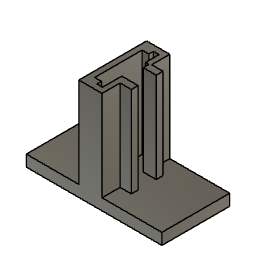
Camera_holder (Autodesk Fusion 360 design; units mm, degrees)
Autodesk Fusion 360 part; units mm, degrees
sketch "Esquisse1" plane through (0, 0, 0) normal (0, 0, 1) x (1, 0, 0)
  line L0 (-29.5177, 14.6047) -> (30.4823, 14.6047)
  line L1 (30.4823, 14.6047) -> (30.4823, -15.3953)
  line L2 (30.4823, -15.3953) -> (-29.5177, -15.3953)
  line L3 (-29.5177, -15.3953) -> (-29.5177, 14.6047)
  dimension "d1" = 60
  dimension "d2" = 30
  constraint horizontal L0
  constraint vertical L1
  constraint horizontal L2
  constraint vertical L3
  measures "d1" distance of L0.start L0.end
  measures "d2" distance of L0.start L2.end
extrude "Extrusion1" add sketch "Esquisse1" along normal blind 5 makes body 1
copy_body "CopyPasteBodies2" bodies 1 makes body 2
move_body "Déplacer2" bodies 2 to x (0, 0, 1) y (0, 1, 0) z (-1, 0, 0) at (40.4823, 0, 29.5177)
move_body "Déplacer3" bodies 2 to x (1, 0, 0) y (0, 1, 0) z (0, 0, 1) at (-35, 0, 5)
extrude "Extrusion2" cut 1 faces at (3.8156, 4.6047, 65) along direction (0, 0, -1) blind 20 on bodies 2 bodies 2
move_body "Aligner1" bodies 1 to x (1, 0, 0) y (0, 1, 0) z (0, 0, 1) at (30, 0, 0)
move_body "Déplacer4" bodies 2 to x (1, 0, 0) y (0, 1, 0) z (0, 0, 1) at (29.5, 0, 0)
move_body "Déplacer5" bodies 2 to x (1, 0, 0) y (0, 1, 0) z (0, 0, 1) at (-29.5, 0, 0)
move_body "Déplacer6" bodies 2 to x (1, 0, 0) y (0, 1, 0) z (0, 0, 1) at (25, 0, 0)
move_body "Déplacer7" bodies 2 to x (1, 0, 0) y (0, 1, 0) z (0, 0, 1) at (2.5, 0, 0)
sketch "Esquisse6" plane through (0, -15.3953, 0) normal (0, -1, 0) x (1, 0, 0)
  line L0 (32.9823, 45) -> (27.9823, 45)
  line L1 (27.9823, 45) -> (27.9823, 5)
  line L2 (27.9823, 5) -> (32.9823, 5)
  line L3 (32.9823, 5) -> (32.9823, 45)
  line L4 (29.2323, 45) -> (31.7323, 45)
  line L5 (31.7323, 45) -> (31.7323, 5)
  line L6 (31.7323, 5) -> (29.2323, 5)
  line L7 (29.2323, 5) -> (29.2323, 45)
  dimension "d7" = 2.5
  dimension "d8" = 1.25
  constraint horizontal L4
  constraint vertical L5
  constraint horizontal L6
  constraint vertical L7
  constraint coincident L2 L5.end
  constraint coincident L0 L4.start
  measures "d7" distance of L4.start L4.end
  measures "d8" distance of L1 L7
extrude "Extrusion3" cut sketch "Esquisse6" against normal up to surface (25 mm away) from surface at -2.5 contours L0 L2 L4 L5 L6 L7 bodies 2
sketch "Esquisse7" plane through (32.9823, 0, 0) normal (1, 0, 0) x (0, 1, 0)
  line L0 (14.6047, 45) -> (-15.3953, 45)
  line L1 (-15.3953, 45) -> (-15.3953, 5)
  line L2 (-15.3953, 5) -> (14.6047, 5)
  line L3 (14.6047, 5) -> (14.6047, 45)
  line L4 (-4.3953, 45) -> (3.6047, 45)
  line L5 (3.6047, 45) -> (3.6047, 5)
  line L6 (3.6047, 5) -> (-4.3953, 5)
  line L7 (-4.3953, 5) -> (-4.3953, 45)
  dimension "d13" = 8
  dimension "d14" = 11
  constraint horizontal L4
  constraint vertical L5
  constraint horizontal L6
  constraint vertical L7
  constraint coincident L0 L4.start
  measures "d13" distance of L4.start L4.end
  measures "d14" distance of L3 L5
extrude "Extrusion4" cut sketch "Esquisse7" against normal blind 2 contours L0 L2 L4 L5 L6 L7 bodies 2
extrude "Extrusion5" add 2 faces at (32.9823, -11.7286, 18.3333) (32.9823, 10.938, 18.3333) along direction (1, 0, 0) blind 1 on bodies 2 bodies 2 1
extrude "Extrusion6" add 1 faces at (27.9823, -5.3953, 31.6667) along direction (-1, 0, 0) blind 1 on bodies 2 bodies 2
sketch "Esquisse11" plane through (31.7323, 0, 0) normal (-1, 0, 0) x (0, -1, 0)
  line L0 (-3.6047, 5) -> (-3.6047, 45)
  line L1 (-3.6047, 45) -> (-12.1047, 45)
  line L2 (-12.1047, 45) -> (-12.1047, 5)
  line L3 (-12.1047, 5) -> (-3.6047, 5)
  line L4 (-3.6047, 45) -> (-6.1047, 45)
  line L5 (-6.1047, 45) -> (-6.1047, 5)
  line L6 (-6.1047, 5) -> (-3.6047, 5)
  line L7 (-3.6047, 5) -> (-3.6047, 45)
  dimension "d24" = 2.5
  dimension "d25" = 40
  constraint horizontal L4
  constraint vertical L5
  constraint horizontal L6
  constraint vertical L7
  constraint coincident L0.end L1.start
  measures "d24" distance of L0.end L4.end
  measures "d25" distance of L4.end L5.end
extrude "Extrusion7" cut sketch "Esquisse11" against normal blind 1.5 contours L0 L1 L3 L4 L5 L6 L7 bodies 2
extrude "Extrusion9" add 1 faces at (26.9823, -5.3953, 31.6667) along direction (-1, 0, 0) blind 2 on bodies 2 bodies 2
sketch "Esquisse13" plane through (29.2323, 0, 0) normal (1, 0, 0) x (0, 1, 0)
  line L0 (12.1047, 5) -> (12.1047, 45)
  line L1 (12.1047, 45) -> (-12.8953, 45)
  line L2 (-12.8953, 45) -> (-12.8953, 5)
  line L3 (-12.8953, 5) -> (12.1047, 5)
  line L4 (-10.8953, 45) -> (10.1047, 45)
  line L5 (10.1047, 45) -> (10.1047, 5)
  line L6 (10.1047, 5) -> (-10.8953, 5)
  line L7 (-10.8953, 5) -> (-10.8953, 45)
  line L8 (14.6047, 5) -> (14.6047, 45)
  dimension "d35" = 21
  dimension "d36" = 4.5
  dimension "d37" = 40
  constraint horizontal L4
  constraint vertical L5
  constraint horizontal L6
  constraint vertical L7
  constraint coincident L1 L4.start
  measures "d35" distance of L4.start L4.end
  measures "d36" distance of L5 L8
  measures "d37" distance of L4.end L5.end
extrude "Extrusion10" cut sketch "Esquisse13" against normal blind 3 contours L1 L3 L4 L5 L6 L7 bodies 2
extrude "Extrusion11" add 1 faces at (24.9823, -5.3953, 31.6667) along direction (-1, 0, 0) blind 1.25 on bodies 2 bodies 2
sketch "Esquisse14" plane through (0, 0, 5) normal (0, 0, 1) x (-1, 0, 0)
  line L0 (-33.9823, -3.6047) -> (-33.2323, -3.6047)
  line L1 (-33.2323, -3.6047) -> (-33.2323, -6.1047)
  line L2 (-33.2323, -6.1047) -> (-31.7323, -6.1047)
  line L3 (-31.7323, -6.1047) -> (-31.7323, -12.1047)
  line L4 (-31.7323, -12.1047) -> (-29.2323, -12.1047)
  line L5 (-29.2323, -12.1047) -> (-29.2323, -10.1047)
  line L6 (-29.2323, -10.1047) -> (-26.2323, -10.1047)
  line L7 (-26.2323, -10.1047) -> (-26.2323, 10.8953)
  line L8 (-26.2323, 10.8953) -> (-29.2323, 10.8953)
  line L9 (-29.2323, 10.8953) -> (-29.2323, 12.8953)
  line L10 (-29.2323, 12.8953) -> (-31.7323, 12.8953)
  line L11 (-31.7323, 12.8953) -> (-31.7323, 4.3953)
  line L12 (-31.7323, 4.3953) -> (-33.9823, 4.3953)
  line L13 (-33.9823, 4.3953) -> (-33.9823, 15.3953)
  line L14 (-33.9823, 15.3953) -> (-60.4823, 15.3953)
  line L15 (-60.4823, 15.3953) -> (-60.4823, -14.6047)
  line L16 (-60.4823, -14.6047) -> (-33.9823, -14.6047)
  line L17 (-33.9823, -14.6047) -> (-33.9823, -3.6047)
  line L18 (-33.9823, 4.3953) -> (-38.9823, 4.3953)
  line L19 (-38.9823, 4.3953) -> (-38.9823, 7.3953)
  line L20 (-38.9823, 7.3953) -> (-33.9823, 7.3953)
  line L21 (-33.9823, 7.3953) -> (-33.9823, 4.3953)
  line L22 (-33.9823, -3.6047) -> (-38.9823, -3.6047)
  line L23 (-38.9823, -3.6047) -> (-38.9823, -6.6047)
  line L24 (-38.9823, -6.6047) -> (-33.9823, -6.6047)
  line L25 (-33.9823, -6.6047) -> (-33.9823, -3.6047)
  dimension "d43" = 5
  dimension "d44" = 3
  dimension "d45" = 5
  dimension "d46" = 3
  constraint horizontal L18
  constraint vertical L19
  constraint horizontal L20
  constraint vertical L21
  constraint coincident L12.end L13.start
  constraint horizontal L22
  constraint vertical L23
  constraint horizontal L24
  constraint vertical L25
  constraint coincident L0.start L17.end
  measures "d43" distance of L19.end L20.end
  measures "d44" distance of L18.end L19.end
  measures "d45" distance of L23.end L24.end
  measures "d46" distance of L22.end L23.end
extrude "Extrusion12" add sketch "Esquisse14" along normal blind 40 contours L17 L22 L23 L24 L25 | L13 L18 L19 L20 L21 bodies 2
